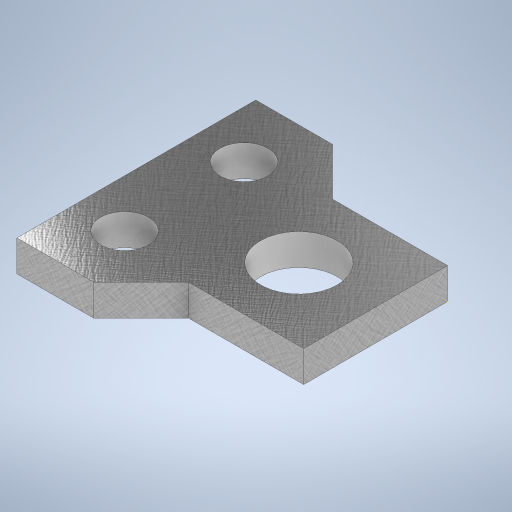
# Autodesk Inventor part: union_movllantas
Saved by Autodesk Inventor 2024 (Build 280153000, 153)
## iProperties
Created: 2023-05-07
Part Number: union_movllantas
Material: Generic
Document SubType Name: Modeling
Designer: Diego
Density: 1 g/cm^3
Appearance: Default
Author: Diego
Autodesk Inventor part; units mm, degrees
ref_plane "YZ Plane" through (0, 0, 0) normal (1, 0, 0) x (0, 1, 0)
ref_plane "XZ Plane" through (0, 0, 0) normal (0, 1, 0) x (-1, 0, 0)
ref_plane "XY Plane" through (0, 0, 0) normal (0, 0, 1) x (1, 0, 0)
sketch "Sketch1" plane through (0, 0, 0) normal (0, 1, 0) x (-1, 0, 0)
  point P0 (0, 0)
sketch "Sketch2" plane through (0, 0, 0) normal (0, 1, 0) x (-1, 0, 0)
  line L0 (0, 0) -> (0, 15)
  line L1 (0, 15) -> (12, 15)
  line L2 (12, 15) -> (16.9497, 19.9497)
  line L3 (12, 15) -> (19, 15) construction
  line L4 (16.9497, 19.9497) -> (24.9497, 19.9497)
  line L5 (0, 7.5) -> (15.5, 7.5) construction
  line L6 (0, 0) -> (12, 0)
  line L7 (12, 0) -> (16.9497, -4.9497)
  line L8 (12, 0) -> (19, 0) construction
  line L9 (16.9497, -4.9497) -> (24.9497, -4.9497)
  line L10 (24.9497, 19.9497) -> (24.9497, -4.9497)
  line L11 (0, 7.5) -> (8, 7.5) construction
  circle A0 centre (8, 7.5) radius 4
  line L12 (24.9497, 7.5) -> (19.9497, 7.5) construction
  line L13 (19.9497, 7.5) -> (19.9497, 19.9497) construction
  circle A1 centre (19.9497, 13.7249) radius 2.5
  line L14 (19.9497, 7.5) -> (19.9497, -4.9497) construction
  circle A2 centre (19.9497, 1.2751) radius 2.5
  dimension "d2" = 15
  dimension "d3" = 12
  dimension "d4" = 7
  dimension "d5" = 45
  dimension "d6" = 8
  dimension "d9" = 8
  dimension "d10" = 8
  dimension "d11" = 5
  dimension "d12" = 5
  constraints: 30 end point, 6 symmetric about line, 5 horizontal, 3 centre point, 3 midpoint, 2 point on line, 2 vertical, 1 coincident, 1 equal length, 1 perpendicular, 1 other
  measures "d2" distance of L0.start L0.end
  measures "d3" distance of L0.end L1.end
  measures "d4" distance of L1.end L2.end
  measures "d5" angle of L3 L2
  measures "d6" distance of L2.end L4.end
  measures "d9" distance of L5.start L11.end
  measures "d10" diameter of A0
  measures "d11" distance of L12.start L12.end
  measures "d12" diameter of A1
extrude "Extrusion1" add sketch "Sketch2" along normal blind 3.25 contours L0 L1 L2 L4 L10 L9 L7 L6 | A0 | A1 | A2
extrude "Extrusion2" cut sketch "Sketch2" along normal blind 3.25 contours A0 | A1 | A2
body "Solid1"
